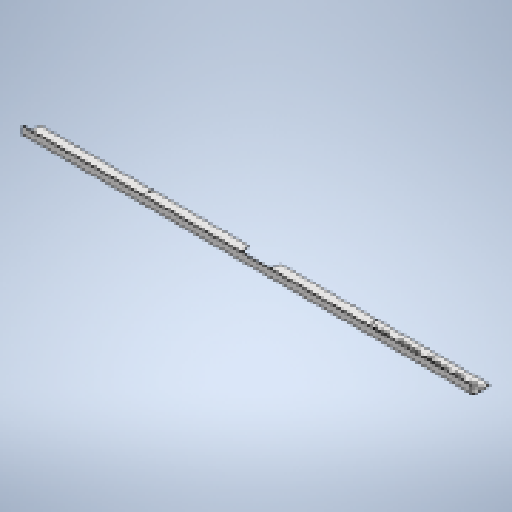
# Autodesk Inventor part: MSC 319 stringer BOARD  ###
Saved by Autodesk Inventor 2025 (Build 290162010, 162A)
## iProperties
Created: 2024-04-28
Part Number: MSC 319 stringer BOARD  ###
Material: Stainless Steel
Document SubType Name: Sheet Metal
Designer: pokla
Stock Number: МОО 308 стрингер борт ###
Mass: 899.514 g
Surface Area: 1167.89 cm^2
Volume: 112.439 cm^3
Density: 8 g/cm^3
Flat Pattern Width: 5.5202 cm
Flat Pattern Length: 11.942 cm
Flat Pattern Area: 65.9224 cm^2
Sheet Metal Rule: AISI304 2mm Die16
Sheet Metal Width: 55,202 mm
Sheet Metal Length: 119,420 mm
Sheet Metal Area: 6592,238 mm^2
Appearance: Default
Author: admin
Autodesk Inventor part; units mm, degrees
ref_plane "YZ Plane" through (0, 0, 0) normal (1, 0, 0) x (0, 1, 0)
ref_plane "XZ Plane" through (0, 0, 0) normal (0, 1, 0) x (-1, 0, 0)
ref_plane "XY Plane" through (0, 0, 0) normal (0, 0, 1) x (1, 0, 0)
sketch "Sketch1" plane through (0, 0, 0) normal (0, 0, 1) x (1, 0, 0)
  line L0 (-490, 39) -> (490, 39)
  line L1 (490, 39) -> (490, 0)
  line L2 (490, 0) -> (-490, 0)
  line L3 (-490, 0) -> (-490, 39)
  point P0 (0, 0)
  point P1 (0, 0)
  dimension "d0" = 980
  dimension "d1" = 39
  measures "d0" distance of L1.end L2.end
  measures "d1" distance of L0.end L1.end
extrude "Plate1" add sketch "Sketch1" along normal blind 2
sketch "Sketch2" plane through (490, 2, 0) normal (0, -1, 0) x (1, 0, 0)
  line L0 (-980, 0) -> (0, 0)
  line L1 (0, 0) -> (0, 20)
  line L2 (0, 20) -> (-980, 20)
  line L3 (-980, 20) -> (-980, 0)
  constraints: 6 end point, 1 horizontal, 1 perpendicular, 1 vertical
edge flange "Flange1" height 20 angle 90 thickness 2 bend radius 2.75 thickness toward (0, -1, 0) relief round relief width 2 relief depth 1 edges at (0, 0, 2) wall of the first edge with corners at (-490, 2, 0) (490, 2, 0) (490, 2, 20) (-490, 2, 20)
bend "Bend1"
corner "Corner1"
sketch "Sketch5" plane through (0, 0, 0) normal (0, 0, -1) x (-1, 0, 0)
  line L0 (490, 39) -> (-490, 39) projected
  line L1 (490, 0) -> (-490, 0) projected
  circle A0 centre (0, 39) radius 35
  line L2 (243.95, 39) -> (246.05, 39)
  line L3 (246.05, 39) -> (246.05, 29)
  line L4 (246.05, 29) -> (243.95, 29)
  line L5 (243.95, 29) -> (243.95, 39)
  line L6 (-243.95, 39) -> (-246.05, 39)
  line L7 (-246.05, 39) -> (-246.05, 29)
  line L8 (-246.05, 29) -> (-243.95, 29)
  line L9 (-243.95, 29) -> (-243.95, 39)
  line L10 (0, 39) -> (0, 0) construction
  circle A1 centre (-490, 39) radius 35
  point P0 (0, 0)
  point P1 (245, 29)
  point P2 (-245, 29)
  point P3 (246.05, 39)
  point P4 (-35, 39)
  point P5 (35, 39)
  point P6 (-246.05, 39)
  dimension "d45" = 70
  dimension "d48" = 2.1
  dimension "d49" = 490
  dimension "d51" = 29
  dimension "d52" = 10
  constraints: 18 end point, 4 midpoint, 4 parallel, 3 perpendicular, 2 centre point, 2 collinear, 2 horizontal, 2 point on line, 1 coincident, 1 equal radius, 1 other
  measures "d45" diameter of A0
  measures "d48" distance of L7.end L8.end
  measures "d49" distance of point (245, 29) point (-245, 29)
  measures "d51" distance between parallel lines of L8 L1
  measures "d52" distance between parallel lines of L0 L8
extrude "Extrusion1" cut sketch "Sketch5" against normal through all contours L3 L4 L5 L0 | L9 L8 L7 L0 | A0 L0 | A1 picked at (-5.9248, 20.8306)
sketch "Sketch9" plane through (0, 0, 2) normal (0, 0, 1) x (1, 0, 0)
  line L0 (485.6141, 29.596) -> (485.6141, 17.596) construction
  line L1 (485.6141, 17.596) -> (285.6141, 17.596) construction
  line L2 (285.6141, 17.596) -> (285.6141, 29.596) construction
  line L3 (285.6141, 29.596) -> (485.6141, 29.596) construction
  line L4 (-490, 39) -> (490, 39) projected
  point P0 (0, 0)
  point P1 (1.05, 68)
  point P2 (490, 39)
  dimension "d40" = 200
  dimension "d41" = 12
  constraints: 1 horizontal, 3 other
  measures "d40" distance of L0.end L1.end
  measures "d41" distance of L1.end L2.end
mark "Mark2"
sketch "Sketch10" plane through (-490, 0, 20) normal (0, -1, 0) x (1, 0, 0)
  line L0 (0, -20) -> (0, -18) projected
  line L1 (0, 0) -> (980, 0) projected
  line L2 (0, -20) -> (884.4148, -20)
  line L3 (884.4148, -20) -> (884.4148, 0)
  line L4 (884.4148, 0) -> (0, 0)
  line L5 (0, 0) -> (0, -20)
  line L6 (884.4148, 0) -> (860.5797, -20)
  point P0 (490, -20)
  dimension "d53" = 50
  dimension "d54" = 884.4148
  constraints: 10 end point, 2 parallel, 2 point on line, 1 horizontal, 1 perpendicular
  measures "d53" angle of L3 L6
  measures "d54" distance between parallel lines of L5 L3
extrude "Extrusion4" cut sketch "Sketch10" against normal through all contours L0 L5 L1 L6 L2
equation "\"d2\" = Thickness"
equation "\"GapSize\" = Thickness"
equation "\"MinimumRemnant\" = 2 * Thickness"
equation "\"BendReliefDepth\" = 0.5 * Thickness"
equation "\"BendReliefWidth\" = Thickness"
equation "\"CornerReliefSize\" = 4 * Thickness"
equation "\"JacobiRadiusSize\" = BendRadius"
equation "\"TransitionRadius\" = BendRadius"
equation "\"d3\" = BendReliefWidth"
equation "\"d4\" = BendReliefDepth"
equation "\"d5\" = MinimumRemnant"
equation "\"d6\" = TransitionRadius"
equation "\"d9\" = BendRadius"
equation "\"d10\" = CornerReliefSize"
equation "\"d11\" = GapSize"
equation "\"d12\" = JacobiRadiusSize"
equation "\"Thickness\" = 2"
equation "\"BendRadius\" = 2.75"
body "Solid1"
